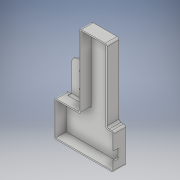
# Autodesk Inventor part: RemoteCase
Saved by Autodesk Inventor 2018 (Build 220112000, 112)
## iProperties
Created: 2020-10-23
Part Number: RemoteCase
Material: Generic
Document SubType Name: Modeling
Designer: dangl
Density: 1 g/cm^3
Appearance: Default
Author: dangl
Autodesk Inventor part; units mm, degrees
ref_plane "YZ Plane" through (0, 0, 0) normal (1, 0, 0) x (0, 1, 0)
ref_plane "XZ Plane" through (0, 0, 0) normal (0, 1, 0) x (-1, 0, 0)
ref_plane "XY Plane" through (0, 0, 0) normal (0, 0, 1) x (1, 0, 0)
sketch "Sketch1" plane through (0, 0, 0) normal (0, 0, 1) x (1, 0, 0)
  line L0 (-5, 110) -> (33, 110)
  line L1 (33, 110) -> (33, 3)
  line L2 (-5, 3) -> (-5, 110)
  line L3 (43, 0) -> (43, -50)
  line L4 (43, -50) -> (-43, -50)
  line L5 (-43, -50) -> (-43, 0)
  line L6 (-43, 0) -> (-8, 0)
  line L7 (36, 0) -> (43, 0)
  line L8 (-4, 112) -> (32, 112)
  line L9 (35, 109) -> (35, 5)
  line L10 (38, 2) -> (42, 2)
  line L11 (45, -1) -> (45, -49)
  line L12 (42, -52) -> (-42, -52)
  line L13 (-45, -49) -> (-45, -1)
  line L14 (-42, 2) -> (-38, 2)
  line L15 (-7, 58) -> (-7, 109)
  arc A0 (-10, 2) -> (-7, 5) centre (-10, 5) ccw
  arc A1 (-42, 2) -> (-45, -1) centre (-42, -1) ccw
  arc A2 (45, -1) -> (42, 2) centre (42, -1) ccw
  arc A3 (42, -52) -> (45, -49) centre (42, -49) ccw
  arc A4 (-45, -49) -> (-42, -52) centre (-42, -49) ccw
  arc A5 (-4, 112) -> (-7, 109) centre (-4, 109) ccw
  arc A6 (35, 109) -> (32, 112) centre (32, 109) ccw
  arc A7 (35, 5) -> (38, 2) centre (38, 5) ccw
  arc A8 (-8, 0) -> (-5, 3) centre (-8, 3) ccw
  arc A9 (33, 3) -> (36, 0) centre (36, 3) ccw
  line L16 (-25, 55) -> (-10, 55)
  line L17 (-7, 55) -> (-7, 5)
  line L18 (-35, 5) -> (-35, 45)
  arc A10 (-25, 55) -> (-35, 45) centre (-25, 45) ccw
  arc A11 (-10, 55) -> (-7, 58) centre (-10, 58) ccw
  arc A12 (-38, 2) -> (-35, 5) centre (-38, 5) ccw
  line L19 (-38, 2) -> (-10, 2)
  line L20 (-7, 58) -> (-7, 55)
  point P0 (0, 0)
  dimension "d1" = 38
  dimension "d2" = 5
  dimension "d4" = 86
  dimension "d5" = 43
  dimension "d6" = 50
  dimension "d7" = 110
  dimension "d8" = 2
  dimension "d9" = 3
  dimension "d10" = 3
  dimension "d11" = 3
  dimension "d13" = 10
  dimension "d14" = 10
  dimension "d15" = 55
  dimension "d16" = 10
  dimension "d17" = 3
  dimension "d18" = 3
  constraints: 42 end point, 27 point on circle, 27 tangent, 13 centre point, 9 parallel, 7 equal radius, 7 perpendicular, 5 horizontal, 3 point on line, 1 vertical, 7 other
  measures "d1" distance of L0.start L0.end
  measures "d2" distance from line of point (0, 0) L2
  measures "d4" distance of L3.end L4.end
  measures "d5" distance from line of point (0, 0) L3
  measures "d6" distance of L4.end L5.end
  measures "d7" distance from line of point (0, 0) L0
  measures "d8" distance between parallel lines of L2 L15
  measures "d9" radius of A0
  measures "d10" radius of A1
  measures "d11" radius of A8
  measures "d13" distance between parallel lines of L13 L18
  measures "d14" distance between parallel lines of L11 L9
  measures "d15" distance from line of point (0, 0) L16
  measures "d16" radius of A10
  measures "d17" radius of A11
  measures "d18" radius of A12
extrude "Extrusion1" add sketch "Sketch1" against normal blind 2 contours L0 L1 A9 L7 L3 L4 L5 L6 A8 L2 | L8 A6 L9 A7 L10 A2 L11 A3 L12 A4 L13 A1 L14 L19 A0 L17 L20 L15 A5 | L20 L17 A0 L19 A12 L18 A10 L16 A11
extrude "Extrusion2" add sketch "Sketch1" along normal blind 16 contours L8 A6 L9 A7 L10 A2 L11 A3 L12 A4 L13 A1 L14 L19 A0 L17 L20 L15 A5
sketch "Sketch2" plane through (45, -49, -2) normal (1, 0, 0) x (0, 0, -1)
  line L0 (-17, 12) -> (-11, 12)
  line L1 (-10, 13) -> (-10, 25)
  line L2 (-11, 26) -> (-18, 26)
  line L3 (-18, 26) -> (-18, 12)
  line L4 (0, 0) -> (-18, 0) projected
  line L5 (0, 48) -> (0, 0) projected
  arc A0 (-11, 12) -> (-10, 13) centre (-11, 13) ccw
  arc A1 (-10, 25) -> (-11, 26) centre (-11, 25) ccw
  arc A2 (-17, 12) -> (-18, 11) centre (-17, 11) ccw
  arc A3 (-18, 26) -> (-18, 26) centre (-18, 27) ccw
  line L6 (-18, 26) -> (-18, 26)
  line L7 (-18, 0) -> (-18, 48) projected
  line L8 (-18, 12) -> (-18, 11)
  point P0 (-2, 49)
  point P1 (-10, 26)
  point P2 (-10, 12)
  dimension "d25" = 14
  dimension "d26" = 26
  dimension "d28" = 10
  dimension "d29" = 1
  dimension "d30" = 1
  dimension "d31" = 1
  constraints: 12 end point, 8 point on circle, 7 tangent, 6 point on line, 4 centre point, 2 parallel, 1 collinear, 1 equal radius, 1 horizontal, 1 perpendicular, 1 vertical
  measures "d25" distance of point (-10, 12) point (-10, 26)
  measures "d26" distance between parallel lines of L4 L2
  measures "d28" distance between parallel lines of L5 L1
  measures "d29" radius of A0
  measures "d30" radius of A2
  measures "d31" radius of A3
extrude "Extrusion3" cut sketch "Sketch2" against normal blind 16 contours A2 L7 L3 L2 A1 L1 A0 L0
sketch "Sketch3" plane through (0, 0, 0) normal (0, 0, 1) x (1, 0, 0)
  circle A0 centre (-22, 40) radius 1.75
  circle A1 centre (-22, 16) radius 1.75
  point P0 (0, 0)
  dimension "d34" = 3.5
  dimension "d35" = 3.5
  dimension "d36" = 24
  dimension "d37" = 16
  dimension "d38" = 22
  dimension "d39" = 22
  constraints: 2 centre point
  measures "d34" diameter of A0
  measures "d35" diameter of A1
  measures "d36" distance of A1.centre A0.centre
  measures "d37" vertical distance of point (0, 0) A1.centre
  measures "d38" horizontal distance of point (0, 0) A1.centre
  measures "d39" horizontal distance of point (0, 0) A0.centre
extrude "Extrusion4" cut sketch "Sketch3" against normal up to next
fillet "Fillet1" radius 3 3 edges at (-7.8787, 2.8787, 0) (-24, 2, 0) (-7, 31.5, 0)
equation "\"d5\" = 0.5 * d4"
equation "\"d7\" = d3"
equation "\"d13\" = d14"
equation "\"d15\" = 0.5 * d7"
equation "\"d39\" = d38"
equation "\"d3\" = 110"
body "Solid1"
